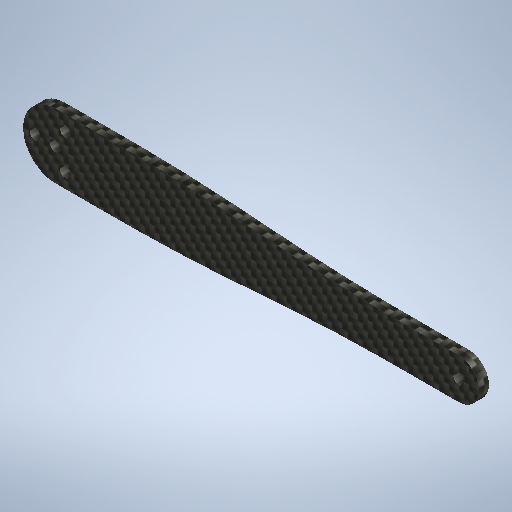
# Autodesk Inventor part: RT_ARM_MC_002
Saved by Autodesk Inventor 2025.3 (Build 293356000, 356)
## iProperties
Created: 2026-04-27
Part Number: RT_ARM_MC_002
Material: CFRP
Document SubType Name: Modeling
Designer: louis
Density: 1.43 g/cm^3
Appearance: Carbon Fiber 1
Author: louis
Autodesk Inventor part; units mm, degrees
ref_plane "YZ Plane" through (0, 0, 0) normal (1, 0, 0) x (0, 1, 0)
ref_plane "XZ Plane" through (0, 0, 0) normal (0, 1, 0) x (-1, 0, 0)
ref_plane "XY Plane" through (0, 0, 0) normal (0, 0, 1) x (1, 0, 0)
sketch "Sketch2" plane through (0, 0, 0) normal (0, 1, 0) x (-1, 0, 0)
  circle A0 centre (0, 0) radius 16
  circle A1 centre (-200, 0) radius 10
  line L0 (0, 0) -> (-200, 0)
  line L1 (0, 16) -> (-20, 16)
  line L2 (-200, 10) -> (-180, 10)
  spline S0 degree 4 poles (-20, 16) (-40.0211, 16) (-80.0633, 16) (-119.9367, 10) (-159.9789, 10) (-180, 10) knots 0 0 0 0 0 0.5 1 1 1 1 1
  line L3 (0, 0) -> (0, 16) construction
  line L4 (-200, 0) -> (-200, 10) construction
  line L5 (0, -16) -> (-20, -16)
  line L6 (-200, -10) -> (-180, -10)
  spline S1 degree 4 poles (-20, -16) (-40.0211, -16) (-80.0633, -16) (-119.9367, -10) (-159.9789, -10) (-180, -10) knots 0 0 0 0 0 0.5 1 1 1 1 1
  line L7 (0, 0) -> (10, 0) construction
  point P0 (0, -16)
  point P1 (-5, 8.6603)
  point P2 (-5, -8.6603)
  dimension "d0" = 32
  dimension "d1" = 20
  dimension "d2" = 200
  dimension "d3" = 20
  dimension "d4" = 20
  dimension "d26" = 10
  dimension "d29" = 360
  constraints: 16 end point, 8 horizontal, 6 coincident, 4 symmetric about line, 2 vertical, 14 other
  measures "d2" distance of L0.start L0.end
  measures "d3" distance of L1.start L1.end
  measures "d4" distance of L2.start L2.end
  measures "d26" distance of L7.start L7.end
extrude "Extrusion1" add sketch "Sketch2" along normal blind 5
hole "Hole1" at (-10, 0, 0) at (5, 0, 8.6603) at (5, 0, -8.6603) direction (0, 1, 0) diameter 5.5 end through all clearance for "Socket Head Cap Screw" size "M5" standard "Ansi Metric M Profile"
hole "Hole2" at (200, 0, 0) at (0, 0, 0) direction (0, 1, 0) diameter 5.5 end through all clearance for "Socket Head Cap Screw" size "M5" standard "Ansi Metric M Profile"
body "Solid1"
